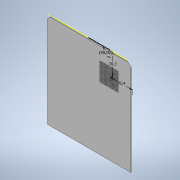
# Autodesk Inventor part: klapa
Saved by Autodesk Inventor 2020 (Build 240168000, 168)
## iProperties
Created: 2019-11-16
Part Number: klapa
Material: Ogólny
Document SubType Name: Modeling
Designer: Hubert Słomion
Density: 1 g/cm^3
Appearance: Domyślna
Author: Hubert Słomion
Autodesk Inventor part; units mm, degrees
ref_plane "YZ Plane" through (0, 0, 0) normal (1, 0, 0) x (0, 1, 0)
ref_plane "XZ Plane" through (0, 0, 0) normal (0, 1, 0) x (-1, 0, 0)
ref_plane "XY Plane" through (0, 0, 0) normal (0, 0, 1) x (1, 0, 0)
sketch "Szkic1" plane through (0, 0, 0) normal (0, 0, 1) x (1, 0, 0)
  line L0 (0, 0) -> (265, 0)
  line L1 (265, 0) -> (265, -300)
  line L2 (265, -300) -> (0, -300)
  line L3 (0, -300) -> (0, 0)
  dimension "d0" = 265
  dimension "d1" = 300
  constraints: 8 end point, 2 parallel, 1 horizontal, 1 perpendicular
  measures "d0" distance of L1.end L2.end
  measures "d1" distance of L0.end L1.end
extrude "Wyciągnięcie proste1" add sketch "Szkic1" along normal blind 4.9
chamfer "Faza2" distance 3 angle 45 4 edges at (132.5, 0, 0) (265, -150, 0) (0, -150, 0) (132.5, -300, 0)
chamfer "Faza3" distance 10 angle 45 2 edges at (1.5, -1.5, 1.5) (263.5, -1.5, 1.5)
sketch "Szkic2" plane through (0, 0, 0) normal (0, 0, -1) x (-1, 0, 0)
  line L0 (-265.2372, -89.5754) -> (-194.8372, -89.5754) construction
  line L1 (-194.8372, 0) -> (-194.8372, -139.5081) construction
  point P0 (0, 0)
  dimension "d13" = 70.4
  constraints: 4 end point, 1 horizontal, 1 vertical
  measures "d13" distance of L0.start L0.end
sketch "Szkic3" plane through (0, 0, 0) normal (0, 0, -1) x (-1, 0, 0)
  line L0 (-12.2474, 0) -> (-252.7526, 0) projected
  line L1 (-195.0449, 0) -> (-124.7449, 0)
  line L2 (-195.0449, 0) -> (-195.0449, -70.3)
  line L3 (-195.0449, 0) -> (-124.7449, 0) construction
  point P0 (0, 0)
  dimension "d15" = 70.3
  dimension "d16" = 90
  constraints: 6 end point, 2 point on line, 1 horizontal, 1 perpendicular, 1 vertical
  measures "d15" distance of L1.start L2.end
  measures "d16" angle of L2 L3
sketch "Szkic5" plane through (0, 0, 0) normal (0, 0, -1) x (-1, 0, 0)
  circle A0 centre (-224.0841, -41.6331) radius 0.875
  line L0 (-195.0449, 0) -> (-195.0449, -70.3) projected
  line L1 (-265.2372, -89.5754) -> (-194.8372, -89.5754) construction
  circle A1 centre (-224.0841, -44.6331) radius 0.875
  circle A2 centre (-224.0841, -47.6331) radius 0.875
  circle A3 centre (-224.0841, -50.6331) radius 0.875
  circle A4 centre (-224.0841, -53.6331) radius 0.875
  circle A5 centre (-224.0841, -56.6331) radius 0.875
  circle A6 centre (-224.0841, -59.6331) radius 0.875
  circle A7 centre (-224.0841, -62.6331) radius 0.875
  circle A8 centre (-224.0841, -65.6331) radius 0.875
  circle A9 centre (-224.0841, -68.6331) radius 0.875
  circle A10 centre (-224.0841, -71.6331) radius 0.875
  circle A11 centre (-224.0841, -74.6331) radius 0.875
  circle A12 centre (-224.0841, -77.6331) radius 0.875
  circle A13 centre (-224.0841, -80.6331) radius 0.875
  circle A14 centre (-224.0841, -83.6331) radius 0.875
  circle A15 centre (-224.0841, -86.6331) radius 0.875
  circle A16 centre (-224.0841, -89.6331) radius 0.875
  circle A17 centre (-224.0841, -92.6331) radius 0.875
  circle A18 centre (-224.0841, -95.6331) radius 0.875
  circle A19 centre (-224.0841, -98.6331) radius 0.875
  circle A20 centre (-221.0841, -41.6331) radius 0.875
  circle A21 centre (-221.0841, -44.6331) radius 0.875
  circle A22 centre (-221.0841, -47.6331) radius 0.875
  circle A23 centre (-221.0841, -50.6331) radius 0.875
  circle A24 centre (-221.0841, -53.6331) radius 0.875
  circle A25 centre (-221.0841, -56.6331) radius 0.875
  circle A26 centre (-221.0841, -59.6331) radius 0.875
  circle A27 centre (-221.0841, -62.6331) radius 0.875
  circle A28 centre (-221.0841, -65.6331) radius 0.875
  circle A29 centre (-221.0841, -68.6331) radius 0.875
  circle A30 centre (-221.0841, -71.6331) radius 0.875
  circle A31 centre (-221.0841, -74.6331) radius 0.875
  circle A32 centre (-221.0841, -77.6331) radius 0.875
  circle A33 centre (-221.0841, -80.6331) radius 0.875
  circle A34 centre (-221.0841, -83.6331) radius 0.875
  circle A35 centre (-221.0841, -86.6331) radius 0.875
  circle A36 centre (-221.0841, -89.6331) radius 0.875
  circle A37 centre (-221.0841, -92.6331) radius 0.875
  circle A38 centre (-221.0841, -95.6331) radius 0.875
  circle A39 centre (-221.0841, -98.6331) radius 0.875
  circle A40 centre (-218.0841, -41.6331) radius 0.875
  circle A41 centre (-218.0841, -44.6331) radius 0.875
  circle A42 centre (-218.0841, -47.6331) radius 0.875
  circle A43 centre (-218.0841, -50.6331) radius 0.875
  circle A44 centre (-218.0841, -53.6331) radius 0.875
  circle A45 centre (-218.0841, -56.6331) radius 0.875
  circle A46 centre (-218.0841, -59.6331) radius 0.875
  circle A47 centre (-218.0841, -62.6331) radius 0.875
  circle A48 centre (-218.0841, -65.6331) radius 0.875
  circle A49 centre (-218.0841, -68.6331) radius 0.875
  circle A50 centre (-218.0841, -71.6331) radius 0.875
  circle A51 centre (-218.0841, -74.6331) radius 0.875
  circle A52 centre (-218.0841, -77.6331) radius 0.875
  circle A53 centre (-218.0841, -80.6331) radius 0.875
  circle A54 centre (-218.0841, -83.6331) radius 0.875
  circle A55 centre (-218.0841, -86.6331) radius 0.875
  circle A56 centre (-218.0841, -89.6331) radius 0.875
  circle A57 centre (-218.0841, -92.6331) radius 0.875
  circle A58 centre (-218.0841, -95.6331) radius 0.875
  circle A59 centre (-218.0841, -98.6331) radius 0.875
  circle A60 centre (-215.0841, -41.6331) radius 0.875
  circle A61 centre (-215.0841, -44.6331) radius 0.875
  circle A62 centre (-215.0841, -47.6331) radius 0.875
  circle A63 centre (-215.0841, -50.6331) radius 0.875
  circle A64 centre (-215.0841, -53.6331) radius 0.875
  circle A65 centre (-215.0841, -56.6331) radius 0.875
  circle A66 centre (-215.0841, -59.6331) radius 0.875
  circle A67 centre (-215.0841, -62.6331) radius 0.875
  circle A68 centre (-215.0841, -65.6331) radius 0.875
  circle A69 centre (-215.0841, -68.6331) radius 0.875
  circle A70 centre (-215.0841, -71.6331) radius 0.875
  circle A71 centre (-215.0841, -74.6331) radius 0.875
  circle A72 centre (-215.0841, -77.6331) radius 0.875
  circle A73 centre (-215.0841, -80.6331) radius 0.875
  circle A74 centre (-215.0841, -83.6331) radius 0.875
  circle A75 centre (-215.0841, -86.6331) radius 0.875
  circle A76 centre (-215.0841, -89.6331) radius 0.875
  circle A77 centre (-215.0841, -92.6331) radius 0.875
  circle A78 centre (-215.0841, -95.6331) radius 0.875
  circle A79 centre (-215.0841, -98.6331) radius 0.875
  circle A80 centre (-212.0841, -41.6331) radius 0.875
  circle A81 centre (-212.0841, -44.6331) radius 0.875
  circle A82 centre (-212.0841, -47.6331) radius 0.875
  circle A83 centre (-212.0841, -50.6331) radius 0.875
  circle A84 centre (-212.0841, -53.6331) radius 0.875
  circle A85 centre (-212.0841, -56.6331) radius 0.875
  circle A86 centre (-212.0841, -59.6331) radius 0.875
  circle A87 centre (-212.0841, -62.6331) radius 0.875
  circle A88 centre (-212.0841, -65.6331) radius 0.875
  circle A89 centre (-212.0841, -68.6331) radius 0.875
  circle A90 centre (-212.0841, -71.6331) radius 0.875
  circle A91 centre (-212.0841, -74.6331) radius 0.875
  circle A92 centre (-212.0841, -77.6331) radius 0.875
  circle A93 centre (-212.0841, -80.6331) radius 0.875
  circle A94 centre (-212.0841, -83.6331) radius 0.875
  circle A95 centre (-212.0841, -86.6331) radius 0.875
  circle A96 centre (-212.0841, -89.6331) radius 0.875
  circle A97 centre (-212.0841, -92.6331) radius 0.875
  circle A98 centre (-212.0841, -95.6331) radius 0.875
  circle A99 centre (-212.0841, -98.6331) radius 0.875
  circle A100 centre (-209.0841, -41.6331) radius 0.875
  circle A101 centre (-209.0841, -44.6331) radius 0.875
  circle A102 centre (-209.0841, -47.6331) radius 0.875
  circle A103 centre (-209.0841, -50.6331) radius 0.875
  circle A104 centre (-209.0841, -53.6331) radius 0.875
  circle A105 centre (-209.0841, -56.6331) radius 0.875
  circle A106 centre (-209.0841, -59.6331) radius 0.875
  circle A107 centre (-209.0841, -62.6331) radius 0.875
  circle A108 centre (-209.0841, -65.6331) radius 0.875
  circle A109 centre (-209.0841, -68.6331) radius 0.875
  circle A110 centre (-209.0841, -71.6331) radius 0.875
  circle A111 centre (-209.0841, -74.6331) radius 0.875
  circle A112 centre (-209.0841, -77.6331) radius 0.875
  circle A113 centre (-209.0841, -80.6331) radius 0.875
  circle A114 centre (-209.0841, -83.6331) radius 0.875
  circle A115 centre (-209.0841, -86.6331) radius 0.875
  circle A116 centre (-209.0841, -89.6331) radius 0.875
  circle A117 centre (-209.0841, -92.6331) radius 0.875
  circle A118 centre (-209.0841, -95.6331) radius 0.875
  circle A119 centre (-209.0841, -98.6331) radius 0.875
  circle A120 centre (-206.0841, -41.6331) radius 0.875
  circle A121 centre (-206.0841, -44.6331) radius 0.875
  circle A122 centre (-206.0841, -47.6331) radius 0.875
  circle A123 centre (-206.0841, -50.6331) radius 0.875
  circle A124 centre (-206.0841, -53.6331) radius 0.875
  circle A125 centre (-206.0841, -56.6331) radius 0.875
  circle A126 centre (-206.0841, -59.6331) radius 0.875
  circle A127 centre (-206.0841, -62.6331) radius 0.875
  circle A128 centre (-206.0841, -65.6331) radius 0.875
  circle A129 centre (-206.0841, -68.6331) radius 0.875
  circle A130 centre (-206.0841, -71.6331) radius 0.875
  circle A131 centre (-206.0841, -74.6331) radius 0.875
  circle A132 centre (-206.0841, -77.6331) radius 0.875
  circle A133 centre (-206.0841, -80.6331) radius 0.875
  circle A134 centre (-206.0841, -83.6331) radius 0.875
  circle A135 centre (-206.0841, -86.6331) radius 0.875
  circle A136 centre (-206.0841, -89.6331) radius 0.875
  circle A137 centre (-206.0841, -92.6331) radius 0.875
  circle A138 centre (-206.0841, -95.6331) radius 0.875
  circle A139 centre (-206.0841, -98.6331) radius 0.875
  circle A140 centre (-203.0841, -41.6331) radius 0.875
  circle A141 centre (-203.0841, -44.6331) radius 0.875
  circle A142 centre (-203.0841, -47.6331) radius 0.875
  circle A143 centre (-203.0841, -50.6331) radius 0.875
  circle A144 centre (-203.0841, -53.6331) radius 0.875
  circle A145 centre (-203.0841, -56.6331) radius 0.875
  circle A146 centre (-203.0841, -59.6331) radius 0.875
  circle A147 centre (-203.0841, -62.6331) radius 0.875
  circle A148 centre (-203.0841, -65.6331) radius 0.875
  circle A149 centre (-203.0841, -68.6331) radius 0.875
  circle A150 centre (-203.0841, -71.6331) radius 0.875
  circle A151 centre (-203.0841, -74.6331) radius 0.875
  circle A152 centre (-203.0841, -77.6331) radius 0.875
  circle A153 centre (-203.0841, -80.6331) radius 0.875
  circle A154 centre (-203.0841, -83.6331) radius 0.875
  circle A155 centre (-203.0841, -86.6331) radius 0.875
  circle A156 centre (-203.0841, -89.6331) radius 0.875
  circle A157 centre (-203.0841, -92.6331) radius 0.875
  circle A158 centre (-203.0841, -95.6331) radius 0.875
  circle A159 centre (-203.0841, -98.6331) radius 0.875
  circle A160 centre (-200.0841, -41.6331) radius 0.875
  circle A161 centre (-200.0841, -44.6331) radius 0.875
  circle A162 centre (-200.0841, -47.6331) radius 0.875
  circle A163 centre (-200.0841, -50.6331) radius 0.875
  circle A164 centre (-200.0841, -53.6331) radius 0.875
  circle A165 centre (-200.0841, -56.6331) radius 0.875
  circle A166 centre (-200.0841, -59.6331) radius 0.875
  circle A167 centre (-200.0841, -62.6331) radius 0.875
  circle A168 centre (-200.0841, -65.6331) radius 0.875
  circle A169 centre (-200.0841, -68.6331) radius 0.875
  circle A170 centre (-200.0841, -71.6331) radius 0.875
  circle A171 centre (-200.0841, -74.6331) radius 0.875
  circle A172 centre (-200.0841, -77.6331) radius 0.875
  circle A173 centre (-200.0841, -80.6331) radius 0.875
  circle A174 centre (-200.0841, -83.6331) radius 0.875
  circle A175 centre (-200.0841, -86.6331) radius 0.875
  circle A176 centre (-200.0841, -89.6331) radius 0.875
  circle A177 centre (-200.0841, -92.6331) radius 0.875
  circle A178 centre (-200.0841, -95.6331) radius 0.875
  circle A179 centre (-200.0841, -98.6331) radius 0.875
  circle A180 centre (-197.0841, -41.6331) radius 0.875
  circle A181 centre (-197.0841, -44.6331) radius 0.875
  circle A182 centre (-197.0841, -47.6331) radius 0.875
  circle A183 centre (-197.0841, -50.6331) radius 0.875
  circle A184 centre (-197.0841, -53.6331) radius 0.875
  circle A185 centre (-197.0841, -56.6331) radius 0.875
  circle A186 centre (-197.0841, -59.6331) radius 0.875
  circle A187 centre (-197.0841, -62.6331) radius 0.875
  circle A188 centre (-197.0841, -65.6331) radius 0.875
  circle A189 centre (-197.0841, -68.6331) radius 0.875
  circle A190 centre (-197.0841, -71.6331) radius 0.875
  circle A191 centre (-197.0841, -74.6331) radius 0.875
  circle A192 centre (-197.0841, -77.6331) radius 0.875
  circle A193 centre (-197.0841, -80.6331) radius 0.875
  circle A194 centre (-197.0841, -83.6331) radius 0.875
  circle A195 centre (-197.0841, -86.6331) radius 0.875
  circle A196 centre (-197.0841, -89.6331) radius 0.875
  circle A197 centre (-197.0841, -92.6331) radius 0.875
  circle A198 centre (-197.0841, -95.6331) radius 0.875
  circle A199 centre (-197.0841, -98.6331) radius 0.875
  circle A200 centre (-194.0841, -41.6331) radius 0.875
  circle A201 centre (-194.0841, -44.6331) radius 0.875
  circle A202 centre (-194.0841, -47.6331) radius 0.875
  circle A203 centre (-194.0841, -50.6331) radius 0.875
  circle A204 centre (-194.0841, -53.6331) radius 0.875
  circle A205 centre (-194.0841, -56.6331) radius 0.875
  circle A206 centre (-194.0841, -59.6331) radius 0.875
  circle A207 centre (-194.0841, -62.6331) radius 0.875
  circle A208 centre (-194.0841, -65.6331) radius 0.875
  circle A209 centre (-194.0841, -68.6331) radius 0.875
  circle A210 centre (-194.0841, -71.6331) radius 0.875
  circle A211 centre (-194.0841, -74.6331) radius 0.875
  circle A212 centre (-194.0841, -77.6331) radius 0.875
  circle A213 centre (-194.0841, -80.6331) radius 0.875
  circle A214 centre (-194.0841, -83.6331) radius 0.875
  circle A215 centre (-194.0841, -86.6331) radius 0.875
  circle A216 centre (-194.0841, -89.6331) radius 0.875
  circle A217 centre (-194.0841, -92.6331) radius 0.875
  circle A218 centre (-194.0841, -95.6331) radius 0.875
  circle A219 centre (-194.0841, -98.6331) radius 0.875
  circle A220 centre (-191.0841, -41.6331) radius 0.875
  circle A221 centre (-191.0841, -44.6331) radius 0.875
  circle A222 centre (-191.0841, -47.6331) radius 0.875
  circle A223 centre (-191.0841, -50.6331) radius 0.875
  circle A224 centre (-191.0841, -53.6331) radius 0.875
  circle A225 centre (-191.0841, -56.6331) radius 0.875
  circle A226 centre (-191.0841, -59.6331) radius 0.875
  circle A227 centre (-191.0841, -62.6331) radius 0.875
  circle A228 centre (-191.0841, -65.6331) radius 0.875
  circle A229 centre (-191.0841, -68.6331) radius 0.875
  circle A230 centre (-191.0841, -71.6331) radius 0.875
  circle A231 centre (-191.0841, -74.6331) radius 0.875
  circle A232 centre (-191.0841, -77.6331) radius 0.875
  circle A233 centre (-191.0841, -80.6331) radius 0.875
  circle A234 centre (-191.0841, -83.6331) radius 0.875
  circle A235 centre (-191.0841, -86.6331) radius 0.875
  circle A236 centre (-191.0841, -89.6331) radius 0.875
  circle A237 centre (-191.0841, -92.6331) radius 0.875
  circle A238 centre (-191.0841, -95.6331) radius 0.875
  circle A239 centre (-191.0841, -98.6331) radius 0.875
  circle A240 centre (-188.0841, -41.6331) radius 0.875
  circle A241 centre (-188.0841, -44.6331) radius 0.875
  circle A242 centre (-188.0841, -47.6331) radius 0.875
  circle A243 centre (-188.0841, -50.6331) radius 0.875
  circle A244 centre (-188.0841, -53.6331) radius 0.875
  circle A245 centre (-188.0841, -56.6331) radius 0.875
  circle A246 centre (-188.0841, -59.6331) radius 0.875
  circle A247 centre (-188.0841, -62.6331) radius 0.875
  circle A248 centre (-188.0841, -65.6331) radius 0.875
  circle A249 centre (-188.0841, -68.6331) radius 0.875
  circle A250 centre (-188.0841, -71.6331) radius 0.875
  circle A251 centre (-188.0841, -74.6331) radius 0.875
  circle A252 centre (-188.0841, -77.6331) radius 0.875
  circle A253 centre (-188.0841, -80.6331) radius 0.875
  circle A254 centre (-188.0841, -83.6331) radius 0.875
  circle A255 centre (-188.0841, -86.6331) radius 0.875
  circle A256 centre (-188.0841, -89.6331) radius 0.875
  circle A257 centre (-188.0841, -92.6331) radius 0.875
  circle A258 centre (-188.0841, -95.6331) radius 0.875
  circle A259 centre (-188.0841, -98.6331) radius 0.875
  circle A260 centre (-185.0841, -41.6331) radius 0.875
  circle A261 centre (-185.0841, -44.6331) radius 0.875
  circle A262 centre (-185.0841, -47.6331) radius 0.875
  circle A263 centre (-185.0841, -50.6331) radius 0.875
  circle A264 centre (-185.0841, -53.6331) radius 0.875
  circle A265 centre (-185.0841, -56.6331) radius 0.875
  circle A266 centre (-185.0841, -59.6331) radius 0.875
  circle A267 centre (-185.0841, -62.6331) radius 0.875
  circle A268 centre (-185.0841, -65.6331) radius 0.875
  circle A269 centre (-185.0841, -68.6331) radius 0.875
  circle A270 centre (-185.0841, -71.6331) radius 0.875
  circle A271 centre (-185.0841, -74.6331) radius 0.875
  circle A272 centre (-185.0841, -77.6331) radius 0.875
  circle A273 centre (-185.0841, -80.6331) radius 0.875
  circle A274 centre (-185.0841, -83.6331) radius 0.875
  circle A275 centre (-185.0841, -86.6331) radius 0.875
  circle A276 centre (-185.0841, -89.6331) radius 0.875
  circle A277 centre (-185.0841, -92.6331) radius 0.875
  circle A278 centre (-185.0841, -95.6331) radius 0.875
  circle A279 centre (-185.0841, -98.6331) radius 0.875
  circle A280 centre (-182.0841, -41.6331) radius 0.875
  circle A281 centre (-182.0841, -44.6331) radius 0.875
  circle A282 centre (-182.0841, -47.6331) radius 0.875
  circle A283 centre (-182.0841, -50.6331) radius 0.875
  circle A284 centre (-182.0841, -53.6331) radius 0.875
  circle A285 centre (-182.0841, -56.6331) radius 0.875
  circle A286 centre (-182.0841, -59.6331) radius 0.875
  circle A287 centre (-182.0841, -62.6331) radius 0.875
  circle A288 centre (-182.0841, -65.6331) radius 0.875
  circle A289 centre (-182.0841, -68.6331) radius 0.875
  circle A290 centre (-182.0841, -71.6331) radius 0.875
  circle A291 centre (-182.0841, -74.6331) radius 0.875
  circle A292 centre (-182.0841, -77.6331) radius 0.875
  circle A293 centre (-182.0841, -80.6331) radius 0.875
  circle A294 centre (-182.0841, -83.6331) radius 0.875
  circle A295 centre (-182.0841, -86.6331) radius 0.875
  circle A296 centre (-182.0841, -89.6331) radius 0.875
  circle A297 centre (-182.0841, -92.6331) radius 0.875
  circle A298 centre (-182.0841, -95.6331) radius 0.875
  circle A299 centre (-182.0841, -98.6331) radius 0.875
  circle A300 centre (-179.0841, -41.6331) radius 0.875
  circle A301 centre (-179.0841, -44.6331) radius 0.875
  circle A302 centre (-179.0841, -47.6331) radius 0.875
  circle A303 centre (-179.0841, -50.6331) radius 0.875
  circle A304 centre (-179.0841, -53.6331) radius 0.875
  circle A305 centre (-179.0841, -56.6331) radius 0.875
  circle A306 centre (-179.0841, -59.6331) radius 0.875
  circle A307 centre (-179.0841, -62.6331) radius 0.875
  circle A308 centre (-179.0841, -65.6331) radius 0.875
  circle A309 centre (-179.0841, -68.6331) radius 0.875
  circle A310 centre (-179.0841, -71.6331) radius 0.875
  circle A311 centre (-179.0841, -74.6331) radius 0.875
  circle A312 centre (-179.0841, -77.6331) radius 0.875
  circle A313 centre (-179.0841, -80.6331) radius 0.875
  circle A314 centre (-179.0841, -83.6331) radius 0.875
  circle A315 centre (-179.0841, -86.6331) radius 0.875
  circle A316 centre (-179.0841, -89.6331) radius 0.875
  circle A317 centre (-179.0841, -92.6331) radius 0.875
  circle A318 centre (-179.0841, -95.6331) radius 0.875
  circle A319 centre (-179.0841, -98.6331) radius 0.875
  circle A320 centre (-176.0841, -41.6331) radius 0.875
  circle A321 centre (-176.0841, -44.6331) radius 0.875
  circle A322 centre (-176.0841, -47.6331) radius 0.875
  circle A323 centre (-176.0841, -50.6331) radius 0.875
  circle A324 centre (-176.0841, -53.6331) radius 0.875
  circle A325 centre (-176.0841, -56.6331) radius 0.875
  circle A326 centre (-176.0841, -59.6331) radius 0.875
  circle A327 centre (-176.0841, -62.6331) radius 0.875
  circle A328 centre (-176.0841, -65.6331) radius 0.875
  circle A329 centre (-176.0841, -68.6331) radius 0.875
  circle A330 centre (-176.0841, -71.6331) radius 0.875
  circle A331 centre (-176.0841, -74.6331) radius 0.875
  circle A332 centre (-176.0841, -77.6331) radius 0.875
  circle A333 centre (-176.0841, -80.6331) radius 0.875
  circle A334 centre (-176.0841, -83.6331) radius 0.875
  circle A335 centre (-176.0841, -86.6331) radius 0.875
  circle A336 centre (-176.0841, -89.6331) radius 0.875
  circle A337 centre (-176.0841, -92.6331) radius 0.875
  circle A338 centre (-176.0841, -95.6331) radius 0.875
  circle A339 centre (-176.0841, -98.6331) radius 0.875
  circle A340 centre (-173.0841, -41.6331) radius 0.875
  circle A341 centre (-173.0841, -44.6331) radius 0.875
  circle A342 centre (-173.0841, -47.6331) radius 0.875
  circle A343 centre (-173.0841, -50.6331) radius 0.875
  circle A344 centre (-173.0841, -53.6331) radius 0.875
  circle A345 centre (-173.0841, -56.6331) radius 0.875
  circle A346 centre (-173.0841, -59.6331) radius 0.875
  circle A347 centre (-173.0841, -62.6331) radius 0.875
  circle A348 centre (-173.0841, -65.6331) radius 0.875
  circle A349 centre (-173.0841, -68.6331) radius 0.875
  circle A350 centre (-173.0841, -71.6331) radius 0.875
  circle A351 centre (-173.0841, -74.6331) radius 0.875
  circle A352 centre (-173.0841, -77.6331) radius 0.875
  circle A353 centre (-173.0841, -80.6331) radius 0.875
  circle A354 centre (-173.0841, -83.6331) radius 0.875
  circle A355 centre (-173.0841, -86.6331) radius 0.875
  circle A356 centre (-173.0841, -89.6331) radius 0.875
  circle A357 centre (-173.0841, -92.6331) radius 0.875
  circle A358 centre (-173.0841, -95.6331) radius 0.875
  circle A359 centre (-173.0841, -98.6331) radius 0.875
  circle A360 centre (-170.0841, -41.6331) radius 0.875
  circle A361 centre (-170.0841, -44.6331) radius 0.875
  circle A362 centre (-170.0841, -47.6331) radius 0.875
  circle A363 centre (-170.0841, -50.6331) radius 0.875
  circle A364 centre (-170.0841, -53.6331) radius 0.875
  circle A365 centre (-170.0841, -56.6331) radius 0.875
  circle A366 centre (-170.0841, -59.6331) radius 0.875
  circle A367 centre (-170.0841, -62.6331) radius 0.875
  circle A368 centre (-170.0841, -65.6331) radius 0.875
  circle A369 centre (-170.0841, -68.6331) radius 0.875
  circle A370 centre (-170.0841, -71.6331) radius 0.875
  circle A371 centre (-170.0841, -74.6331) radius 0.875
  circle A372 centre (-170.0841, -77.6331) radius 0.875
  circle A373 centre (-170.0841, -80.6331) radius 0.875
  circle A374 centre (-170.0841, -83.6331) radius 0.875
  circle A375 centre (-170.0841, -86.6331) radius 0.875
  circle A376 centre (-170.0841, -89.6331) radius 0.875
  circle A377 centre (-170.0841, -92.6331) radius 0.875
  circle A378 centre (-170.0841, -95.6331) radius 0.875
  circle A379 centre (-170.0841, -98.6331) radius 0.875
  circle A380 centre (-167.0841, -41.6331) radius 0.875
  circle A381 centre (-167.0841, -44.6331) radius 0.875
  circle A382 centre (-167.0841, -47.6331) radius 0.875
  circle A383 centre (-167.0841, -50.6331) radius 0.875
  circle A384 centre (-167.0841, -53.6331) radius 0.875
  circle A385 centre (-167.0841, -56.6331) radius 0.875
  circle A386 centre (-167.0841, -59.6331) radius 0.875
  circle A387 centre (-167.0841, -62.6331) radius 0.875
  circle A388 centre (-167.0841, -65.6331) radius 0.875
  circle A389 centre (-167.0841, -68.6331) radius 0.875
  circle A390 centre (-167.0841, -71.6331) radius 0.875
  circle A391 centre (-167.0841, -74.6331) radius 0.875
  circle A392 centre (-167.0841, -77.6331) radius 0.875
  circle A393 centre (-167.0841, -80.6331) radius 0.875
  circle A394 centre (-167.0841, -83.6331) radius 0.875
  circle A395 centre (-167.0841, -86.6331) radius 0.875
  circle A396 centre (-167.0841, -89.6331) radius 0.875
  circle A397 centre (-167.0841, -92.6331) radius 0.875
  circle A398 centre (-167.0841, -95.6331) radius 0.875
  circle A399 centre (-167.0841, -98.6331) radius 0.875
  point P0 (0, 0)
  point P1 (-221.0841, -41.6331)
  point P2 (-221.0841, -44.6331)
  point P3 (-221.0841, -47.6331)
  point P4 (-221.0841, -50.6331)
  point P5 (-221.0841, -53.6331)
  point P6 (-221.0841, -56.6331)
  point P7 (-221.0841, -59.6331)
  point P8 (-221.0841, -62.6331)
  point P9 (-221.0841, -65.6331)
  point P10 (-221.0841, -68.6331)
  point P11 (-221.0841, -71.6331)
  point P12 (-221.0841, -74.6331)
  point P13 (-221.0841, -77.6331)
  point P14 (-221.0841, -80.6331)
  point P15 (-221.0841, -83.6331)
  point P16 (-221.0841, -86.6331)
  point P17 (-221.0841, -89.6331)
  point P18 (-221.0841, -92.6331)
  point P19 (-221.0841, -95.6331)
  point P20 (-221.0841, -98.6331)
  point P21 (-218.0841, -41.6331)
  point P22 (-218.0841, -44.6331)
  point P23 (-218.0841, -47.6331)
  point P24 (-218.0841, -50.6331)
  point P25 (-218.0841, -53.6331)
  point P26 (-218.0841, -56.6331)
  point P27 (-218.0841, -59.6331)
  point P28 (-218.0841, -62.6331)
  point P29 (-218.0841, -65.6331)
  point P30 (-218.0841, -68.6331)
  point P31 (-218.0841, -71.6331)
  point P32 (-218.0841, -74.6331)
  point P33 (-218.0841, -77.6331)
  point P34 (-218.0841, -80.6331)
  point P35 (-218.0841, -83.6331)
  point P36 (-218.0841, -86.6331)
  point P37 (-218.0841, -89.6331)
  point P38 (-218.0841, -92.6331)
  point P39 (-218.0841, -95.6331)
  point P40 (-218.0841, -98.6331)
  point P41 (-215.0841, -41.6331)
  point P42 (-215.0841, -44.6331)
  point P43 (-215.0841, -47.6331)
  point P44 (-215.0841, -50.6331)
  point P45 (-215.0841, -53.6331)
  point P46 (-215.0841, -56.6331)
  point P47 (-215.0841, -59.6331)
  point P48 (-215.0841, -62.6331)
  point P49 (-215.0841, -65.6331)
  point P50 (-215.0841, -68.6331)
  point P51 (-215.0841, -71.6331)
  point P52 (-215.0841, -74.6331)
  point P53 (-215.0841, -77.6331)
  point P54 (-215.0841, -80.6331)
  point P55 (-215.0841, -83.6331)
  point P56 (-215.0841, -86.6331)
  point P57 (-215.0841, -89.6331)
  point P58 (-215.0841, -92.6331)
  point P59 (-215.0841, -95.6331)
  point P60 (-215.0841, -98.6331)
  point P61 (-212.0841, -41.6331)
  point P62 (-212.0841, -44.6331)
  point P63 (-212.0841, -47.6331)
  point P64 (-212.0841, -50.6331)
  point P65 (-212.0841, -53.6331)
  point P66 (-212.0841, -56.6331)
  point P67 (-212.0841, -59.6331)
  point P68 (-212.0841, -62.6331)
  point P69 (-212.0841, -65.6331)
  point P70 (-212.0841, -68.6331)
  point P71 (-212.0841, -71.6331)
  point P72 (-212.0841, -74.6331)
  point P73 (-212.0841, -77.6331)
  point P74 (-212.0841, -80.6331)
  point P75 (-212.0841, -83.6331)
  point P76 (-212.0841, -86.6331)
  point P77 (-212.0841, -89.6331)
  point P78 (-212.0841, -92.6331)
  point P79 (-212.0841, -95.6331)
  point P80 (-212.0841, -98.6331)
  point P81 (-209.0841, -41.6331)
  point P82 (-209.0841, -44.6331)
  point P83 (-209.0841, -47.6331)
  point P84 (-209.0841, -50.6331)
  point P85 (-209.0841, -53.6331)
  point P86 (-209.0841, -56.6331)
  point P87 (-209.0841, -59.6331)
  point P88 (-209.0841, -62.6331)
  point P89 (-209.0841, -65.6331)
  point P90 (-209.0841, -68.6331)
  point P91 (-209.0841, -71.6331)
  point P92 (-209.0841, -74.6331)
  point P93 (-209.0841, -77.6331)
  point P94 (-209.0841, -80.6331)
  point P95 (-209.0841, -83.6331)
  point P96 (-209.0841, -86.6331)
  point P97 (-209.0841, -89.6331)
  point P98 (-209.0841, -92.6331)
  point P99 (-209.0841, -95.6331)
  point P100 (-209.0841, -98.6331)
  point P101 (-206.0841, -41.6331)
  point P102 (-206.0841, -44.6331)
  point P103 (-206.0841, -47.6331)
  point P104 (-206.0841, -50.6331)
  point P105 (-206.0841, -53.6331)
  point P106 (-206.0841, -56.6331)
  point P107 (-206.0841, -59.6331)
  point P108 (-206.0841, -62.6331)
  point P109 (-206.0841, -65.6331)
  point P110 (-206.0841, -68.6331)
  point P111 (-206.0841, -71.6331)
  point P112 (-206.0841, -74.6331)
  point P113 (-206.0841, -77.6331)
  point P114 (-206.0841, -80.6331)
  point P115 (-206.0841, -83.6331)
  point P116 (-206.0841, -86.6331)
  point P117 (-206.0841, -89.6331)
  point P118 (-206.0841, -92.6331)
  point P119 (-206.0841, -95.6331)
  point P120 (-206.0841, -98.6331)
  point P121 (-203.0841, -41.6331)
  point P122 (-203.0841, -44.6331)
  point P123 (-203.0841, -47.6331)
  point P124 (-203.0841, -50.6331)
  point P125 (-203.0841, -53.6331)
  point P126 (-203.0841, -56.6331)
  point P127 (-203.0841, -59.6331)
  point P128 (-203.0841, -62.6331)
  point P129 (-203.0841, -65.6331)
  point P130 (-203.0841, -68.6331)
  point P131 (-203.0841, -71.6331)
  point P132 (-203.0841, -74.6331)
  point P133 (-203.0841, -77.6331)
  point P134 (-203.0841, -80.6331)
  point P135 (-203.0841, -83.6331)
  point P136 (-203.0841, -86.6331)
  point P137 (-203.0841, -89.6331)
  point P138 (-203.0841, -92.6331)
  point P139 (-203.0841, -95.6331)
  point P140 (-203.0841, -98.6331)
  point P141 (-200.0841, -41.6331)
  point P142 (-200.0841, -44.6331)
  point P143 (-200.0841, -47.6331)
  point P144 (-200.0841, -50.6331)
  point P145 (-200.0841, -53.6331)
  point P146 (-200.0841, -56.6331)
  point P147 (-200.0841, -59.6331)
  point P148 (-200.0841, -62.6331)
  point P149 (-200.0841, -65.6331)
  point P150 (-200.0841, -68.6331)
  point P151 (-200.0841, -71.6331)
  point P152 (-200.0841, -74.6331)
  point P153 (-200.0841, -77.6331)
  point P154 (-200.0841, -80.6331)
  point P155 (-200.0841, -83.6331)
  point P156 (-200.0841, -86.6331)
  point P157 (-200.0841, -89.6331)
  point P158 (-200.0841, -92.6331)
  point P159 (-200.0841, -95.6331)
  point P160 (-200.0841, -98.6331)
  point P161 (-197.0841, -41.6331)
  point P162 (-197.0841, -44.6331)
  point P163 (-197.0841, -47.6331)
  point P164 (-197.0841, -50.6331)
  point P165 (-197.0841, -53.6331)
  point P166 (-197.0841, -56.6331)
  point P167 (-197.0841, -59.6331)
  point P168 (-197.0841, -62.6331)
  point P169 (-197.0841, -65.6331)
  point P170 (-197.0841, -68.6331)
  point P171 (-197.0841, -71.6331)
  point P172 (-197.0841, -74.6331)
  point P173 (-197.0841, -77.6331)
  point P174 (-197.0841, -80.6331)
  point P175 (-197.0841, -83.6331)
  point P176 (-197.0841, -86.6331)
  point P177 (-197.0841, -89.6331)
  point P178 (-197.0841, -92.6331)
  point P179 (-197.0841, -95.6331)
  point P180 (-197.0841, -98.6331)
  point P181 (-194.0841, -41.6331)
  point P182 (-194.0841, -44.6331)
  point P183 (-194.0841, -47.6331)
  point P184 (-194.0841, -50.6331)
  point P185 (-194.0841, -53.6331)
  point P186 (-194.0841, -56.6331)
  point P187 (-194.0841, -59.6331)
  point P188 (-194.0841, -62.6331)
  point P189 (-194.0841, -65.6331)
  point P190 (-194.0841, -68.6331)
  point P191 (-194.0841, -71.6331)
  point P192 (-194.0841, -74.6331)
  point P193 (-194.0841, -77.6331)
  point P194 (-194.0841, -80.6331)
  point P195 (-194.0841, -83.6331)
  point P196 (-194.0841, -86.6331)
  point P197 (-194.0841, -89.6331)
  point P198 (-194.0841, -92.6331)
  point P199 (-194.0841, -95.6331)
  dimension "d30" = 1.75
  dimension "d33" = 3
  dimension "d36" = 3
  dimension "d41" = 3
  dimension "d44" = 3
  constraints: 400 centre point, 2 horizontal, 2 vertical, 1197 other
  measures "d30" diameter of A0
  measures "d33" distance of A0.centre point (-224.084, -44.633)
  measures "d36" distance of A0.centre point (-221.084, -41.633)
  measures "d41" distance of A0.centre A1.centre
  measures "d44" distance of A0.centre A20.centre
extrude "Wyciągnięcie proste4" cut sketch "Szkic5" against normal blind 119.25
